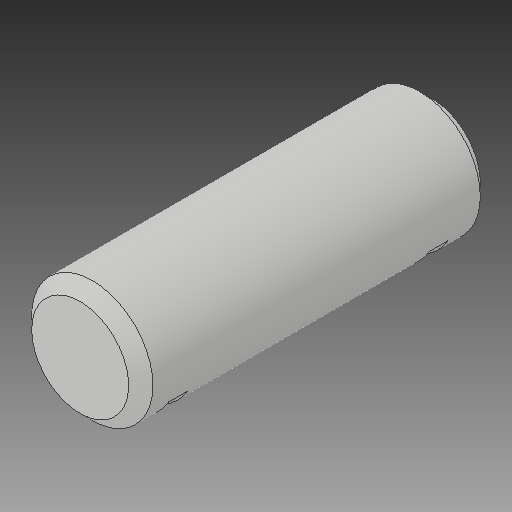
# Autodesk Inventor part: čep
Saved by Autodesk Inventor 2019 (Build 230136000, 136)
## iProperties
Created: 2018-11-24
Part Number: čep
Material: Generic
Document SubType Name: Modeling
Designer: Radek
Density: 1 g/cm^3
Appearance: Default
Author: Radek
Autodesk Inventor part; units mm, degrees
ref_plane "YZ Plane" through (0, 0, 0) normal (1, 0, 0) x (0, 1, 0)
sketch "Náčrt1" plane through (0, 0, 0) normal (0, 1, 0) x (-1, 0, 0)
  line L0 (0, 0) -> (8, 0)
  line L1 (8, 0) -> (10, -2)
  line L2 (10, -2) -> (10, -56)
  line L3 (10, -56) -> (8, -58)
  line L4 (8, -58) -> (0, -58)
  line L5 (0, -58) -> (0, 0)
  dimension "d0" = 20
  dimension "d1" = 58
  dimension "d2" = 2
  dimension "d3" = 2
  dimension "d4" = 2
  constraints: 12 end point, 3 perpendicular, 1 horizontal, 1 parallel
  measures "d0" diameter of L2 L5
  measures "d1" distance between parallel lines of L0 L4
  measures "d2" horizontal distance of L0.end L1.end
  measures "d3" horizontal distance of L0.end L1.end
  measures "d4" horizontal distance of L2.end L3.end
revolve "Rotace1" add sketch "Náčrt1" angle 360 about axis through (0, 0, -58) along (0, 0, 1)
sketch "Náčrt2" plane through (0, 0, -58) normal (0, 0, -1) x (-1, 0, 0)
  point P0 (0, 0)
  point P1 (0, 0)
  constraints: 1 coincident
hole "Díra1" at (0, 0, -58) direction (0, 0, 1) diameter 3 depth 35 tip angle 118
sketch "Náčrt4" plane through (0, 0, -58) normal (0, 0, -1) x (-1, 0, 0)
  point P0 (0, 0)
  point P1 (0, 0)
  constraints: 1 coincident
hole "Díra2" at (0, 0, -58) direction (0, 0, 1) diameter 6 depth 7 tip angle 59
ref_plane "Pracovní rovina1" through (0, -10, 0) normal (0, 1, 0) x (-1, 0, 0)
sketch "Náčrt6" plane through (0, -10, 0) normal (0, 1, 0) x (-1, 0, 0)
  line L0 (-8, -58) -> (8, -58) projected
  line L1 (10, -2) -> (10, -56) projected
  point P0 (0, 0)
  point P1 (0, -28)
  dimension "d21" = 30
  dimension "d22" = 10
  measures "d21" distance from line of L0 point (0, -28)
  measures "d22" distance from line of L1 point (0, -28)
hole "Díra3" at (0, -10, -28) direction (0, 1, 0) diameter 3 depth 10 tip angle 118
ref_plane "Pracovní rovina2" through (0, 0, -28) normal (0, 0, 1) x (1, 0, 0)
sketch "Náčrt7" plane through (0, 0, -28) normal (0, 0, 1) x (1, 0, 0)
  circle A0 centre (0, 0) radius 10 projected
  arc A1 (1.496, -9.8875) -> (-1.4956, -9.8875) centre (0.0002, -10) ccw
  arc A2 (-1.4956, -9.8875) -> (1.496, -9.8875) centre (0, 0) ccw
  line L0 (0, -14.0017) -> (0, 14.0003) projected
  point P0 (0, 0)
  dimension "d31" = 3
  dimension "d32" = 0.0002
  constraints: 5 point on circle, 2 centre point, 1 coincident, 2 other
  measures "d31" diameter of A1
  measures "d32" distance from line of L0 A1.centre
extrude "Vysunutí1" cut sketch "Náčrt7" along normal mid plane 25 contours A0 L0 A1 | A0 A1 L0 picked at (0.2902, -9.5113) picked at (-0.2901, -9.5113)
sketch "Náčrt8" plane through (0, 0, 0) normal (1, 0, 0) x (0, 1, 0)
  arc A0 (-10, -40.5) -> (-8.5, -34.6905) centre (-20.5, -34.6905) ccw
  line L0 (-10, -2) -> (-10, -56) projected
  line L1 (-10, -40.5) -> (-9.8875, -40.5) projected
  line L2 (-10, -40.5) -> (-8.5, -40.5)
  line L3 (-8.5, -40.5) -> (-8.5, -34.6905)
  line L4 (-26.6, -28) -> (16.1, -28) projected
  arc A1 (-8.5, -21.3095) -> (-10, -15.5) centre (-20.5, -21.3095) ccw
  line L5 (-10, -15.5) -> (-8.5, -15.5)
  line L6 (-8.5, -15.5) -> (-8.5, -21.3095)
  point P0 (0, 0)
  point P1 (-9.8875, -40.5)
  dimension "d35" = 24
  dimension "d36" = 10.5
  dimension "d37" = 12
  constraints: 8 end point, 4 point on circle, 4 symmetric about line, 2 centre point, 1 horizontal, 1 perpendicular, 1 point on line, 1 other
  measures "d35" diameter of A0
  measures "d36" distance from line of L0 A0.centre
  measures "d37" distance from line of A0.centre L3
extrude "Vysunutí2" add sketch "Náčrt8" along normal mid plane 3
sketch "Náčrt10" plane through (0, 0, 0) normal (1, 0, 0) x (0, 1, 0)
  line L0 (-9.8875, -40.2918) -> (-9.8869, -40.2906) projected
  line L1 (-9.8869, -40.2906) -> (-9.8869, -40.5) projected
  line L2 (-9.8869, -40.5) -> (-10, -40.5) projected
  line L3 (-10, -40.5) -> (-9.8869, -40.5) projected
  line L4 (-9.8869, -40.5) -> (-9.8869, -40.2906) projected
  line L5 (-9.8869, -40.2906) -> (-9.8875, -40.2919) projected
  line L6 (-9.8875, -40.2919) -> (-9.8875, -28.1152) projected
  line L7 (-9.8875, -27.8848) -> (-9.8875, -15.7081) projected
  line L8 (-9.8875, -15.7081) -> (-9.8869, -15.7094) projected
  line L9 (-9.8869, -15.7094) -> (-9.8869, -15.5) projected
  line L10 (-9.8869, -15.5) -> (-10, -15.5) projected
  line L11 (-10, -15.5) -> (-9.8869, -15.5) projected
  line L12 (-9.8869, -15.5) -> (-9.8869, -15.7094) projected
  line L13 (-9.8869, -15.7094) -> (-9.8875, -15.7082) projected
  line L14 (-9.8875, -15.7082) -> (-9.8875, -27.8902) projected
  line L15 (-9.8875, -28.1098) -> (-9.8875, -40.2918) projected
  line L16 (-10, -56) -> (10, -56) projected
  line L17 (-10, -2) -> (10, -2) projected
  line L18 (-10, -49) -> (-5, -49)
  line L19 (-5, -49) -> (-5, -52)
  line L20 (-5, -52) -> (-10, -52)
  line L21 (-10, -52) -> (-10, -49)
  line L22 (-10, -2) -> (-10, -56) projected
  line L23 (-8, -58) -> (8, -58) projected
  line L24 (-10, -9) -> (-5, -9)
  line L25 (-5, -9) -> (-5, -6)
  line L26 (-5, -6) -> (-10, -6)
  line L27 (-10, -9) -> (-10, -6)
  point P0 (0, 0)
  dimension "d40" = 0
  dimension "d41" = 5
  dimension "d42" = 3
  dimension "d43" = 6
  dimension "d44" = 3
  dimension "d45" = 40
  dimension "d46" = 5
  constraints: 16 end point, 5 perpendicular, 2 horizontal, 2 point on line, 2 vertical alignment, 1 collinear
  measures "d40" distance between parallel lines of L21 L22
  measures "d41" distance of L19.end L20.end
  measures "d42" distance of L18.end L19.end
  measures "d43" distance between parallel lines of L23 L20
  measures "d44" distance of L24.end L25.end
  measures "d45" distance between parallel lines of L18 L24
  measures "d46" distance of L25.end L26.end
extrude "Vysunutí3" cut sketch "Náčrt10" along normal through all both and the other way through all
